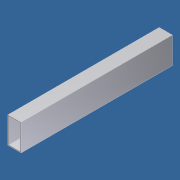
# Autodesk Inventor part: GE-12026-05
Saved by Autodesk Inventor 2012 (Build 160160000, 160)
## iProperties
Created: 2011-10-09
Part Number: GE-12026-05
Document SubType Name: Modeling
Designer: dfoster
Density: 1 g/cm^3
Description: Foot
Material: Default
Title: Foot
Author: dfoster
Autodesk Inventor part; units mm, degrees
ref_plane "YZ Plane" through (0, 0, 0) normal (1, 0, 0) x (0, 1, 0)
ref_plane "XZ Plane" through (0, 0, 0) normal (0, 1, 0) x (-1, 0, 0)
ref_plane "XY Plane" through (0, 0, 0) normal (0, 0, 1) x (1, 0, 0)
sketch "Sketch1" plane through (0, 0, 0) normal (0, 0, 1) x (1, 0, 0)
  line L0 (0, 0) -> (44.45, 0)
  line L1 (44.45, 0) -> (44.45, -88.9)
  line L2 (44.45, -88.9) -> (0, -88.9)
  line L3 (0, -88.9) -> (0, 0)
  line L4 (41.275, -3.175) -> (3.175, -3.175)
  line L5 (3.175, -3.175) -> (3.175, -85.725)
  line L6 (3.175, -85.725) -> (41.275, -85.725)
  line L7 (41.275, -85.725) -> (41.275, -3.175)
  dimension "d0" = 44.45
  dimension "d1" = 88.9
  dimension "d2" = 3.175
  constraints: 16 end point, 4 parallel, 2 perpendicular, 1 horizontal, 3 other
  measures "d0" distance between parallel lines of L1 L3
  measures "d1" distance of L0.end L1.end
  measures "d2" distance between parallel lines of L4 L0
extrude "Extrusion1" add sketch "Sketch1" along normal blind 508
body "Solid1"
